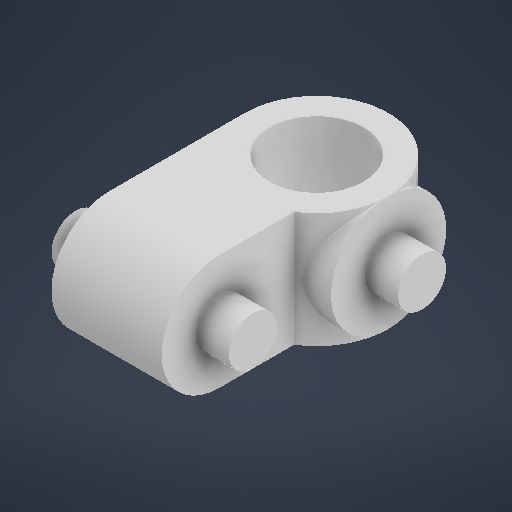
# Autodesk Inventor part: Кулак
Saved by Autodesk Inventor 2026.2 (Build 302298000, 298)
## iProperties
Created: 2026-02-19
Part Number: Кулак
Material: Типовые
Document SubType Name: Modeling
Designer: Leonid
Density: 1 g/cm^3
Appearance: По умолчанию
Author: Leonid
Autodesk Inventor part; units mm, degrees
ref_plane "YZ Plane" through (0, 0, 0) normal (1, 0, 0) x (0, 1, 0)
ref_plane "XZ Plane" through (0, 0, 0) normal (0, 1, 0) x (-1, 0, 0)
ref_plane "XY Plane" through (0, 0, 0) normal (0, 0, 1) x (1, 0, 0)
sketch "Эскиз1" plane through (0, 0, 0) normal (0, 1, 0) x (-1, 0, 0)
  circle A0 centre (0, 0) radius 2.45
  circle A1 centre (0, 0) radius 3.75
  dimension "d0" = 4.9
  dimension "d1" = 7.5
  constraints: 2 centre point, 2 coincident
  measures "d0" diameter of A0
  measures "d1" diameter of A1
extrude "Выдавливание1" add sketch "Эскиз1" along normal blind 6
sketch "Эскиз2" plane through (0, 0, 0) normal (1, 0, 0) x (0, 1, 0)
  circle A0 centre (3, 0) radius 1.25
  line L0 (0, -3.75) -> (0, 3.75) projected
  circle A1 centre (3, 0) radius 3
  circle A2 centre (3, 7.071) radius 1.25
  arc A3 (6, 7.071) -> (0, 7.071) centre (3, 7.071) ccw
  line L1 (3, 0) -> (3, 7.071) construction
  line L2 (6, 0) -> (6, 7.071)
  line L3 (0, 7.071) -> (0, 0)
  point P0 (0, 0)
  dimension "d7" = 6
  dimension "d4" = 2.5
  dimension "d12" = 2.5
  dimension "d13" = 6
  dimension "d14" = 7.071
  constraints: 6 end point, 3 centre point, 3 vertical, 2 coincident, 2 point on circle, 2 tangent, 1 parallel, 3 other
  measures "d4" diameter of A0
  measures "d12" diameter of A2
  measures "d13" diameter of A3
  measures "d14" distance of L1.start L1.end
extrude "Выдавливание3" add sketch "Эскиз2" along normal mid plane 7.5 contours A1
extrude "Выдавливание5" add sketch "Эскиз2" along normal blind 2 and the other way blind 3.75 contours L0 L3 A3 L2 A1
extrude "Выдавливание2" add sketch "Эскиз2" along normal mid plane 11 contours A0
extrude "Выдавливание4" cut sketch "Эскиз1" along normal blind 6 contours A0
extrude "Выдавливание7" add sketch "Эскиз2" along normal blind 3.75 and the other way blind 5.5 contours A2
